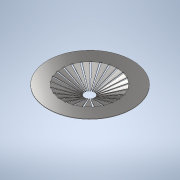
# Autodesk Inventor part: Docisk_Sprężyna_Talerzowa
Saved by Autodesk Inventor 2022 (Build 260153000, 153)
## iProperties
Created: 2021-05-23
Part Number: Docisk_Sprężyna_Talerzowa
Material: Stal, węglowa
Document SubType Name: Modeling
Designer: Matik
Density: 7.85 g/cm^3
Appearance: Częściowo polerowany
Author: Matik
Autodesk Inventor part; units mm, degrees
ref_plane "YZ Plane" through (0, 0, 0) normal (1, 0, 0) x (0, 1, 0)
ref_plane "XY Plane" through (0, 0, 0) normal (0, 0, 1) x (1, 0, 0)
ref_plane "Płaszczyzna konstrukcyjna1" through (0, -1, 0) normal (0, 1, 0) x (-1, 0, 0)
sketch "Szkic2" plane through (0, -1, 0) normal (0, 1, 0) x (-1, 0, 0)
  line L0 (0, 0) -> (-186, 0)
  circle A0 centre (-93, 0) radius 93
  dimension "d4" = 186
  constraints: 2 end point, 1 horizontal, 1 midpoint, 3 other
  measures "d4" distance of L0.start L0.end
extrude "Wyciągnięcie proste1" add sketch "Szkic2" against normal blind 1
sketch "Szkic3" plane through (93, -2, 0) normal (0, -1, 0) x (1, 0, 0)
  circle A0 centre (-1, 0) radius 62
  circle A1 centre (-1, 0) radius 92
  point P0 (-93, 0)
  dimension "d8" = 184
  dimension "d9" = 30
  constraints: 1 centre point, 1 coincident, 1 horizontal alignment, 2 other
extrude "Wyciągnięcie proste2" cut sketch "Szkic3" against normal blind 1 contours A0
ref_plane "Płaszczyzna konstrukcyjna5" through (92, -1, 0) normal (0, 1, 0) x (1, 0, 0)
sketch "Szkic6" plane through (92, -1, 0) normal (0, 1, 0) x (1, 0, 0)
  circle A0 centre (0, 0) radius 62 projected
  line L0 (0, -62) -> (-6, -62)
  line L1 (0, -62) -> (6, -62)
  line L2 (6, -62) -> (6, -61)
  line L3 (-6, -62) -> (-6, -61)
  line L4 (-6, -61) -> (6, -61)
  point P0 (-92, 0)
  point P1 (-6, -61.709)
  point P2 (6, -61.709)
  dimension "d17" = 6
  dimension "d18" = 6
  dimension "d19" = 1
  dimension "d20" = 1
  constraints: 10 end point, 4 horizontal, 1 perpendicular, 1 vertical, 2 other
  measures "d17" distance of L0.start L0.end
  measures "d18" distance of L0.start L1.end
  measures "d19" distance of L1.end L2.end
  measures "d20" distance of L0.end L3.end
extrude "Wyciągnięcie proste4" add sketch "Szkic6" against normal blind 1 contours L3 L4 L2 A0 picked at (0.6676, -61.3225)
ref_plane "Płaszczyzna konstrukcyjna4" through (98, -1, 11) normal (0, 0, -1) x (-1, 0, 0)
sketch "Szkic7" plane through (98, -1, 11) normal (0, 0, -1) x (-1, 0, 0)
  line L0 (6, -21) -> (5.5, -21)
  line L1 (5.5, -21) -> (5.5, -20)
  line L2 (6.5, -20) -> (6.5, -21)
  line L3 (6.5, -21) -> (6, -21)
  line L4 (0, 0) -> (15.998, 0)
  line L5 (0, -2.5111) -> (0, 0)
  line L6 (0, 0) -> (12, 0) projected
  line L7 (0, 0) -> (12, 0) projected
  line L8 (0, 0) -> (0, -1) projected
  line L9 (12, -1) -> (0, -1) projected
  line L10 (12, 0) -> (12, -1) projected
  line L11 (0, 0) -> (0, -1) projected
  line L12 (12, 0) -> (12, -1) projected
  line L13 (6, -1) -> (6, -20)
  line L14 (6.5, -20) -> (6, -20)
  line L15 (6, -20) -> (5.5, -20)
  point P0 (98, 1)
  dimension "d31" = 1
  dimension "d45" = 0.5
  constraints: 18 end point, 3 horizontal, 1 collinear, 1 midpoint, 1 perpendicular, 1 vertical
  measures "d31" distance of L0.end L1.end
  measures "d45" distance of L2.start L14.end
loft "Wyciągnięcie złożone1" add profiles "Szkic7" section 1 edges at (92, -1, 61) (98, -1.5, 61) (92, -2, 61) (86, -1.5, 61) contours L0 L1 L15 L14 L2 L3
pattern_circular "Szyk kołowy2" count 25 over 360 about axis through (92, -2, 0) along (0, 1, 0) of "Wyciągnięcie złożone1", "Wyciągnięcie proste4"
